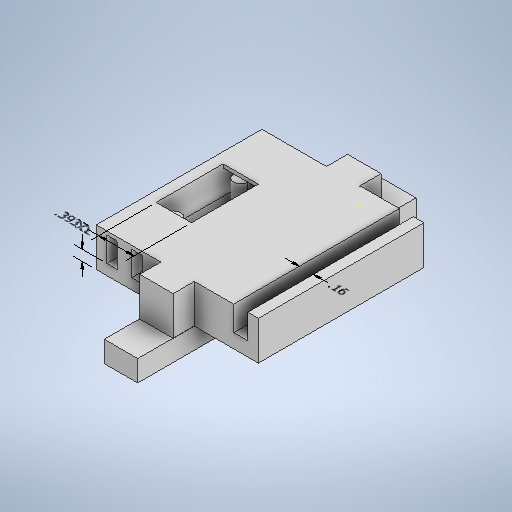
# Autodesk Inventor part: table_bridge
Saved by Autodesk Inventor 2025.2 (Build 292293000, 293)
## iProperties
Created: 2024-12-26
Part Number: table_bridge
Material: Generic
Document SubType Name: Modeling
Designer: holz
Density: 1 g/cm^3
Appearance: Default
Author: holz
Autodesk Inventor part; units mm, degrees
ref_plane "YZ Plane" through (0, 0, 0) normal (1, 0, 0) x (0, 1, 0)
ref_plane "XZ Plane" through (0, 0, 0) normal (0, 1, 0) x (-1, 0, 0)
ref_plane "XY Plane" through (0, 0, 0) normal (0, 0, 1) x (1, 0, 0)
sketch "Sketch1" plane through (0, 0, 0) normal (0, 1, 0) x (-1, 0, 0)
  line L0 (21.9604, 29.5602) -> (-24.0396, 29.5602)
  line L1 (-24.0396, 29.5602) -> (-24.0396, -29.4398)
  line L2 (-24.0396, -29.4398) -> (21.9604, -29.4398)
  line L3 (21.9604, -29.4398) -> (21.9604, 29.5602)
  dimension "d0" = 46
  dimension "d1" = 59
  constraints: 8 end point, 2 parallel, 1 horizontal, 1 perpendicular
  measures "d0" distance of L2.end L1.end
  measures "d1" distance of L1.end L0.end
extrude "Extrusion1" add sketch "Sketch1" along normal blind 11
sketch "Sketch2" plane through (0, 11, 0) normal (0, 1, 0) x (1, 0, 0)
  line L0 (-18.9604, -32.4344) -> (-8.9604, -32.4344)
  line L1 (-8.9604, -32.4344) -> (-8.9604, 37.5656)
  line L2 (-8.9604, 37.5656) -> (-18.9604, 37.5656)
  line L3 (-18.9604, 37.5656) -> (-18.9604, -32.4344)
  line L4 (-21.9604, 29.4398) -> (-21.9604, -29.5602) projected
  point P0 (0, 0)
  dimension "d4" = 10
  dimension "d5" = 70
  dimension "d6" = 3
  constraints: 8 end point, 2 parallel, 1 horizontal, 1 perpendicular
  measures "d4" distance of L2.end L1.end
  measures "d5" distance of L1.end L0.end
  measures "d6" distance between parallel lines of L3 L4
extrude "Extrusion2" cut sketch "Sketch2" against normal blind 8
sketch "Sketch3" plane through (0, 11, 0) normal (0, 1, 0) x (1, 0, 0)
  line L0 (17.0396, -31.142) -> (21.0396, -31.142)
  line L1 (21.0396, -31.142) -> (21.0396, 38.858)
  line L2 (21.0396, 38.858) -> (17.0396, 38.858)
  line L3 (17.0396, 38.858) -> (17.0396, -31.142)
  line L4 (24.0396, -29.5602) -> (24.0396, 29.4398) projected
  point P0 (0, 0)
  dimension "d9" = 4
  dimension "d10" = 70
  dimension "d11" = 3
  constraints: 8 end point, 2 parallel, 1 horizontal, 1 perpendicular
  measures "d9" distance of L2.end L1.end
  measures "d10" distance of L1.end L0.end
  measures "d11" distance between parallel lines of L4 L1
extrude "Extrusion3" cut sketch "Sketch3" against normal blind 7
sketch "Sketch4" plane through (0, 3, 0) normal (0, 1, 0) x (1, 0, 0)
  line L0 (-15.9604, -24.5602) -> (-15.9604, -9.5602)
  line L1 (-11.9604, -24.5602) -> (-11.9604, -9.5602)
  arc A0 (-11.9604, -9.5602) -> (-15.9604, -9.5602) centre (-13.9604, -9.5602) ccw
  arc A1 (-15.9604, -24.5602) -> (-11.9604, -24.5602) centre (-13.9604, -24.5602) ccw
  line L2 (-18.9604, -29.5602) -> (-18.9604, 29.4398) projected
  line L3 (-8.9604, 29.4398) -> (-8.9604, -29.5602) projected
  line L4 (-8.9604, -29.5602) -> (-18.9604, -29.5602) projected
  line L5 (-15.9604, 9.4398) -> (-15.9604, 24.4398)
  line L6 (-11.9604, 9.4398) -> (-11.9604, 24.4398)
  arc A2 (-11.9604, 24.4398) -> (-15.9604, 24.4398) centre (-13.9604, 24.4398) ccw
  arc A3 (-15.9604, 9.4398) -> (-11.9604, 9.4398) centre (-13.9604, 9.4398) ccw
  line L7 (-18.9604, 29.4398) -> (-8.9604, 29.4398) projected
  point P0 (0, 0)
  point P1 (-13.9604, 29.4398)
  point P2 (-11.9604, 16.9398)
  point P3 (-15.9604, 16.9398)
  dimension "d14" = 4
  dimension "d21" = 3
  dimension "d22" = 3
  dimension "d31" = 5
  dimension "d32" = 15
  dimension "d43" = 15
  dimension "d44" = 5
  dimension "d45" = 4
  dimension "d46" = 3
  dimension "d47" = 3
  constraints: 8 end point, 8 point on circle, 8 tangent, 4 centre point, 4 vertical, 3 midpoint
  measures "d14" distance between parallel lines of L1 L0
  measures "d21" distance between parallel lines of L2 L0
  measures "d22" distance between parallel lines of L3 L1
  measures "d31" distance from line of L4 A1.centre
  measures "d32" distance of A0.centre A1.centre
  measures "d43" distance of L5.start L5.end
  measures "d44" distance of point (-13.96, 29.44) A2.centre
  measures "d45" distance of point (-11.96, 16.94) point (-15.96, 16.94)
  measures "d46" distance between parallel lines of L3 L6
  measures "d47" distance between parallel lines of L2 L5
extrude "Extrusion4" add sketch "Sketch4" along normal blind 7 contours L0 A0 L1 A1 | L5 A2 L6 A3
sketch "Sketch6" plane through (0, 10, 0) normal (0, 1, 0) x (1, 0, 0)
  line L0 (-19.9604, -23.5602) -> (-7.9604, -23.5602)
  line L1 (-7.9604, -23.5602) -> (-7.9604, -9.5602)
  line L2 (-7.9604, -9.5602) -> (-19.9604, -9.5602)
  line L3 (-19.9604, -9.5602) -> (-19.9604, -23.5602)
  arc A0 (-11.9604, -9.5602) -> (-15.9604, -9.5602) centre (-13.9604, -9.5602) ccw projected
  line L4 (-15.9604, -9.5602) -> (-15.9604, -24.5602) projected
  line L5 (-18.9604, -29.5602) -> (-18.9604, 29.4398) projected
  line L6 (-8.9604, 29.4398) -> (-8.9604, -29.5602) projected
  line L7 (-19.9604, 9.4398) -> (-19.9604, 23.4398)
  line L8 (-19.9604, 23.4398) -> (-7.9604, 23.4398)
  line L9 (-7.9604, 23.4398) -> (-7.9604, 9.4398)
  line L10 (-7.9604, 9.4398) -> (-19.9604, 9.4398)
  point P0 (0, 0)
  point P1 (-13.9604, -7.5602)
  point P2 (-19.9604, -16.5602)
  point P3 (-7.9604, 16.4398)
  point P4 (-19.9604, 16.4398)
  point P5 (-18.9604, 9.4398)
  point P6 (-8.9604, 9.4398)
  point P7 (-8.9604, 23.4398)
  point P8 (-18.9604, 23.4398)
  dimension "d33" = 14
  dimension "d35" = 0
  dimension "d37" = 1
  dimension "d41" = 12
  dimension "d48" = 14
  dimension "d49" = 12
  dimension "d62" = 19
  constraints: 14 end point, 5 perpendicular, 3 midpoint, 1 parallel, 1 point on circle, 1 vertical, 3 other
  measures "d35" distance from line of A0.centre L2
  measures "d37" distance between parallel lines of L5 L3
  measures "d41" distance between parallel lines of L1 L3
  measures "d48" distance between parallel lines of L8 L10
  measures "d49" distance of point (-7.96, 16.44) point (-19.96, 16.44)
  measures "d62" distance between parallel lines of L10 L2
extrude "Extrusion6" add sketch "Sketch6" along normal blind 1 contours L3 L2 L5 L0 | L5 L2 L4 L0 | L4 L2 L6 L0 | L6 L2 L1 L0 | L5 L8 L6 L10
sketch "Sketch8" plane through (0, 0, 0) normal (0, -1, 0) x (1, 0, 0)
  line L0 (5.7896, 31.0602) -> (-3.7104, 31.0602)
  line L1 (-3.7104, 31.0602) -> (-3.7104, -30.9398)
  line L2 (-3.7104, -30.9398) -> (5.7896, -30.9398)
  line L3 (5.7896, -30.9398) -> (5.7896, 31.0602)
  line L4 (-21.9604, 29.5602) -> (24.0396, 29.5602) projected
  line L5 (24.0396, -29.4398) -> (-21.9604, -29.4398) projected
  line L6 (24.0396, 29.5602) -> (24.0396, -29.4398) projected
  line L7 (-21.9604, -29.4398) -> (-21.9604, 29.5602) projected
  point P0 (0, 0)
  point P1 (-3.7104, -29.4398)
  point P2 (5.7896, -29.4398)
  point P3 (5.7896, 29.5602)
  point P4 (-3.7104, 29.5602)
  dimension "d50" = 9.5
  dimension "d51" = 62
  dimension "d52" = 1.5
  dimension "d53" = 1.5
  dimension "d54" = 18.25
  dimension "d55" = 18.25
  constraints: 8 end point, 2 parallel, 1 horizontal, 1 perpendicular
  measures "d50" distance between parallel lines of L1 L3
  measures "d51" distance between parallel lines of L2 L0
  measures "d52" distance between parallel lines of L4 L0
  measures "d53" distance between parallel lines of L5 L2
  measures "d54" distance between parallel lines of L6 L3
  measures "d55" distance between parallel lines of L7 L1
extrude "Extrusion7" add sketch "Sketch8" along normal blind 6 contours L3 L5 L1 L4
sketch "Sketch9" plane through (24.0396, 0, -29.4398) normal (0, 0, -1) x (-1, 0, 0)
  point P0 (24.0396, 0)
sketch "Sketch10" plane through (24.0396, 0, -29.4398) normal (0, 0, -1) x (-1, 0, 0)
  line L0 (0, 0) -> (18.25, 0) projected
  line L1 (27.75, 0) -> (27.75, -6) projected
  line L2 (18.25, 0) -> (27.75, 0)
  line L3 (27.75, 0) -> (27.75, -6)
  line L4 (27.75, -6) -> (18.25, -6)
  line L5 (18.25, -6) -> (18.25, 0)
  point P0 (24.0396, 0)
  constraints: 8 end point, 2 parallel, 1 horizontal, 1 perpendicular
extrude "Extrusion8" add sketch "Sketch10" along normal blind 10
sketch "Sketch11" plane through (-21.9604, 0, 29.5602) normal (0, 0, 1) x (1, 0, 0)
  line L0 (0, 0) -> (18.25, 0) projected
  line L1 (18.25, 0) -> (27.75, 0)
  line L2 (27.75, 0) -> (27.75, -6)
  line L3 (27.75, -6) -> (18.25, -6)
  line L4 (18.25, -6) -> (18.25, 0)
  point P0 (21.9604, 0)
  constraints: 8 end point, 2 parallel, 1 horizontal, 1 perpendicular
extrude "Extrusion9" add sketch "Sketch11" along normal blind 10
sketch "Sketch12" plane through (0, 11, 0) normal (0, 1, 0) x (1, 0, 0)
  line L0 (24.0396, -29.5602) -> (24.0396, 29.4398) projected
  line L1 (-21.9604, 29.4398) -> (-21.9604, -29.5602) projected
  line L2 (24.0396, -29.5602) -> (-21.9604, -29.5602)
  line L3 (-21.9604, -29.5602) -> (-21.9604, -23.5602)
  line L4 (24.0396, -23.5602) -> (24.0396, -29.5602)
  line L5 (-21.9604, 29.4398) -> (24.0396, 29.4398)
  line L6 (24.0396, 29.4398) -> (24.0396, 23.4398)
  line L7 (-21.9604, 23.4398) -> (-21.9604, 29.4398)
  line L8 (-21.9604, -23.5602) -> (-3.6341, -23.5602)
  line L9 (5.8705, -23.5602) -> (24.0396, -23.5602)
  line L10 (24.0396, 23.4398) -> (5.8705, 23.4398)
  line L11 (-3.6341, 23.4398) -> (-21.9604, 23.4398)
  line L12 (-3.6341, 29.4398) -> (-3.6341, 23.4398)
  line L13 (-3.6341, -23.5602) -> (-3.6341, -29.5602)
  line L14 (5.8705, -29.5602) -> (5.8705, -23.5602)
  line L15 (5.8705, 23.4398) -> (5.8705, 29.4398)
  point P0 (0, 0)
  point P1 (-21.9604, -29.5602)
  dimension "d63" = 6
  dimension "d64" = 6
  constraints: 28 end point, 10 parallel, 6 point on line, 2 horizontal, 2 perpendicular
  measures "d63" distance of L2.end L3.end
  measures "d64" distance of L5.end L6.end
extrude "Extrusion10" cut sketch "Sketch12" against normal blind 100 contours L2 L14 L9 L0 | L10 L15 L5 L0 | L2 L1 L8 L13 | L12 L11 L1 L5
body "Solid1"
